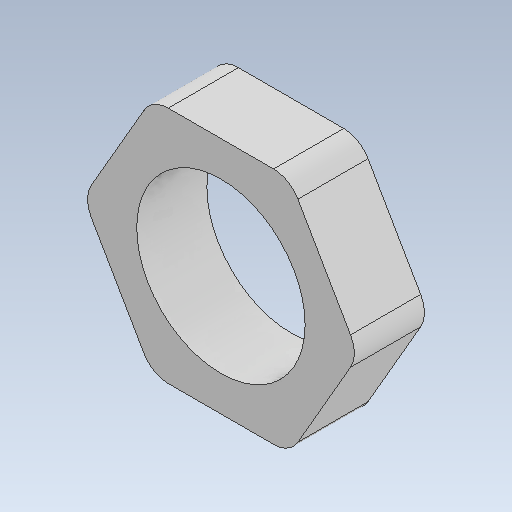
# Autodesk Inventor part: M12_NUT_1.262.1200.50
Saved by Autodesk Inventor 2021 (Build 250183000, 183)
## iProperties
Created: 2020-06-10
Part Number: M12_NUT_1.262.1200.50
Material: Generic
Document SubType Name: Modeling
Designer: lgnds
Density: 1 g/cm^3
Appearance: Default
Author: lgnds
Autodesk Inventor part; units mm, degrees
ref_plane "YZ Plane" through (0, 0, 0) normal (1, 0, 0) x (0, 1, 0)
ref_plane "XZ Plane" through (0, 0, 0) normal (0, 1, 0) x (-1, 0, 0)
ref_plane "XY Plane" through (0, 0, 0) normal (0, 0, 1) x (1, 0, 0)
sketch "Sketch1" plane through (0, 0, 0) normal (0, 0, 1) x (1, 0, 0)
  line L0 (9.815, 0) -> (4.9075, -8.5)
  line L1 (4.9075, -8.5) -> (-4.9075, -8.5)
  line L2 (-4.9075, -8.5) -> (-9.815, 0)
  line L3 (-9.815, 0) -> (-4.9075, 8.5)
  line L4 (-4.9075, 8.5) -> (4.9075, 8.5)
  line L5 (4.9075, 8.5) -> (9.815, 0)
  point P0 (0, 0)
  point P1 (0, 0)
  dimension "d0" = 17
  constraints: 12 end point, 1 coincident, 13 other
  measures "d0" distance between parallel lines of L4 L1
extrude "Extrusion1" add sketch "Sketch1" along normal mid plane 5
sketch "Sketch2" plane through (0, 0, 2.5) normal (0, 0, 1) x (1, 0, 0)
  circle A0 centre (0, 0) radius 6
  dimension "d3" = 12
  constraints: 1 centre point, 1 coincident
  measures "d3" diameter of A0
extrude "Extrusion2" cut sketch "Sketch2" against normal through all
fillet "Fillet1" radius 2 6 edges at (4.9075, -8.5, 0) (-4.9075, -8.5, 0) (-9.815, 0, 0) (-4.9075, 8.5, 0) (4.9075, 8.5, 0) (9.815, 0, 0)
body "Solid1"
